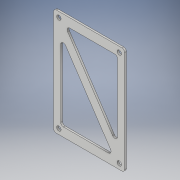
# Autodesk Inventor part: pompression_plate
Saved by Autodesk Inventor 2019 (Build 230136000, 136)
## iProperties
Created: 2019-05-30
Part Number: pompression_plate
Material: Generic
Document SubType Name: Modeling
Designer: steve
Density: 1 g/cm^3
Appearance: Default
Author: steve
Autodesk Inventor part; units mm, degrees
ref_plane "YZ Plane" through (0, 0, 0) normal (1, 0, 0) x (0, 1, 0)
ref_plane "XZ Plane" through (0, 0, 0) normal (0, 1, 0) x (-1, 0, 0)
ref_plane "XY Plane" through (0, 0, 0) normal (0, 0, 1) x (1, 0, 0)
sketch "Sketch1" plane through (0, 0, 0) normal (0, 0, 1) x (1, 0, 0)
  line L0 (-185, -300) -> (185, -300)
  line L1 (200, -285) -> (200, 285)
  line L2 (185, 300) -> (-185, 300)
  line L3 (-200, 285) -> (-200, -285)
  line L4 (-200, -300) -> (200, 300) construction
  line L5 (200, -300) -> (-200, 300) construction
  arc A0 (-185, 300) -> (-200, 285) centre (-185, 285) ccw
  arc A1 (200, 285) -> (185, 300) centre (185, 285) ccw
  arc A2 (185, -300) -> (200, -285) centre (185, -285) ccw
  arc A3 (-200, -285) -> (-185, -300) centre (-185, -285) ccw
  line L6 (-160, -235) -> (-160, 145.389)
  line L7 (-132.5192, 153.7095) -> (121.0734, -226.6795)
  line L8 (108.5926, -250) -> (-145, -250)
  line L9 (-121.0734, 226.6795) -> (132.5192, -153.7095)
  line L10 (160, -145.389) -> (160, 235)
  line L11 (145, 250) -> (-108.5926, 250)
  arc A4 (-132.5192, 153.7095) -> (-160, 145.389) centre (-145, 145.389) ccw
  arc A5 (-108.5926, 250) -> (-121.0734, 226.6795) centre (-108.5926, 235) ccw
  arc A6 (108.5926, -250) -> (121.0734, -226.6795) centre (108.5926, -235) ccw
  arc A7 (132.5192, -153.7095) -> (160, -145.389) centre (145, -145.389) ccw
  arc A8 (160, 235) -> (145, 250) centre (145, 235) ccw
  arc A9 (-160, -235) -> (-145, -250) centre (-145, -235) ccw
  circle A10 centre (-170, 270) radius 12.5
  line L12 (0, -424.3492) -> (0, 424.3492) projected
  line L13 (-284.3492, 0) -> (284.3492, 0) projected
  circle A11 centre (170, 270) radius 12.5
  circle A12 centre (-170, -270) radius 12.5
  circle A13 centre (170, -270) radius 12.5
  point P0 (0, 0)
  dimension "width" = 400
  dimension "depth" = 600
  dimension "outerCornnerRadius" = 15
  dimension "d5" = 15
  dimension "d7" = 50
  dimension "d8" = 50
  dimension "innerCorrerRadius" = 15
  dimension "d14" = 40
  dimension "d15" = 40
  dimension "d16" = 40
  dimension "d17" = 40
  dimension "d20" = 25
  dimension "d21" = 30
  dimension "d22" = 30
  constraints: 24 end point, 20 point on circle, 20 tangent, 14 centre point, 8 point on line, 7 equal radius, 4 parallel, 4 perpendicular, 3 symmetric about line, 2 midpoint, 1 horizontal, 1 vertical, 3 other
  measures "width" distance of L4.end L5.end
  measures "depth" distance of L5.start L4.end
  measures "outerCornnerRadius" radius of A0
  measures "d5" radius of A1
  measures "d7" distance between parallel lines of L0 L8
  measures "d8" distance between parallel lines of L2 L11
  measures "innerCorrerRadius" radius of A4
  measures "d14" distance from line of L5 A6.centre
  measures "d15" distance from line of L5 A4.centre
  measures "d16" distance between parallel lines of L3 L6
  measures "d17" distance between parallel lines of L1 L10
  measures "d20" diameter of A10
  measures "d21" distance from line of L2 A10.centre
  measures "d22" distance from line of L3 A10.centre
extrude "Extrusion3" add sketch "Sketch1" along normal blind 10 contours A3 L3 L13 L6 A9 L8 L12 L0 | L12 L8 A6 L7 L13 L9 A7 L10 L1 A2 L0 | L3 A0 L2 L12 L11 A5 L9 L13 L7 A4 L6 | L7 L13 L12 | L13 L10 A8 L11 L12 L2 A1 L1 | L12 L9 L13
equation "\"d5\" = outerCornnerRadius"
equation "\"d15\" = d14"
body "Solid3"
